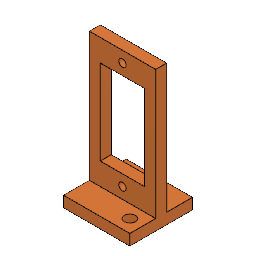
Fixateur servo (Autodesk Fusion 360 design; units mm, degrees)
Autodesk Fusion 360 part; units mm, degrees
sketch "Sketch base" plane through (0, 0, 0) normal (0, 1, 0) x (1, 0, 0)
  line L0 (0, 0) -> (18, 0)
  line L1 (18, 0) -> (18, -3)
  line L2 (18, -3) -> (0, -3)
  line L3 (0, -3) -> (0, 0)
  dimension "d1" = 18
  dimension "d2" = 3
  constraint horizontal L0
  constraint vertical L1
  constraint horizontal L2
  constraint vertical L3
  constraint coincident L0.start L3.end
  measures "d1" distance of L0.start L0.end
  measures "d2" distance of L0.start L2.end
extrude "Extrude base" add sketch "Sketch base" along normal blind 38
sketch "Sketch face" plane through (0, 0, 0) normal (0, 0, -1) x (-1, 0, 0)
  line L0 (-18, 0) -> (0, 0)
  line L1 (0, 0) -> (0, 38)
  line L2 (0, 38) -> (-18, 38)
  line L3 (-18, 38) -> (-18, 0)
  circle A0 centre (-9, 35) radius 1
  circle A1 centre (-9, 6) radius 1
  line L4 (-15, 32) -> (-3, 32)
  line L5 (-3, 32) -> (-3, 9)
  line L6 (-3, 9) -> (-15, 9)
  line L7 (-15, 9) -> (-15, 32)
  line L8 (0, 0) -> (-18, 0)
  line L9 (-18, 0) -> (-18, 3)
  line L10 (-18, 3) -> (0, 3)
  line L11 (0, 3) -> (0, 0)
  dimension "d5" = 2
  dimension "d6" = 2
  dimension "d7" = 12
  dimension "d8" = 3
  dimension "d9" = 3
  dimension "d10" = 3
  dimension "d13" = 3
  dimension "d14" = 9
  dimension "d15" = 9
  dimension "d19" = 3
  dimension "d34" = 23
  constraint horizontal L4
  constraint vertical L5
  constraint horizontal L6
  constraint vertical L7
  constraint horizontal L8
  constraint vertical L9
  constraint horizontal L10
  constraint vertical L11
  constraint coincident L0.end L1.start
  measures "d5" diameter of A0
  measures "d6" diameter of A1
  measures "d7" distance of L4.start L4.end
  measures "d8" distance of L3 L7
  measures "d9" distance of A0.centre L4
  measures "d10" distance of A1.centre L6
  measures "d13" distance of L2 A0.centre
  measures "d14" distance of L1 A0.centre
  measures "d15" distance of L1 A1.centre
  measures "d19" distance of L0.end L10.end
  measures "d34" distance of L4 L6
extrude "Extrude face" cut sketch "Sketch face" against normal blind 4 contours A0 | A1 | L4 L5 L6 L7
extrude "Extrude socle" add sketch "Sketch face" along normal blind 7 and the other way blind 10 contours L0 L1 L3 L8 L9 L10 L11
hole "Hole1" at (3.5, 3, -3.5) direction (0, -1, 0) diameter 3 depth 5 tip angle 180
hole "Hole2" at (14.5, 3, 6.5) direction (0, -1, 0) diameter 3 depth 5 tip angle 180
named bodies: "Fixateur"
